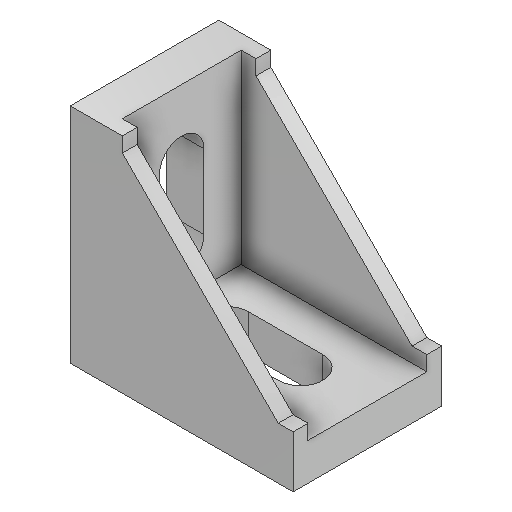
# Autodesk Inventor part: Esquinero
Saved by Autodesk Inventor 2026.1 (Build 301233000, 233)
## iProperties
Created: 2025-06-30
Part Number: Esquinero
Material: Aluminio 6061
Document SubType Name: Modeling
Designer: piero
Density: 2.7 g/cm^3
Appearance: Satinado - Plateado
Author: piero
Autodesk Inventor part; units mm, degrees
ref_plane "YZ Plane" through (0, 0, 0) normal (1, 0, 0) x (0, 1, 0)
ref_plane "XZ Plane" through (0, 0, 0) normal (0, 1, 0) x (-1, 0, 0)
ref_plane "XY Plane" through (0, 0, 0) normal (0, 0, 1) x (1, 0, 0)
sketch "Boceto1" plane through (0, 0, 0) normal (1, 0, 0) x (0, 1, 0)
  line L0 (0, 0) -> (30, 0)
  line L1 (30, 0) -> (30, -20)
  line L2 (30, -20) -> (0, -20)
  line L3 (0, -20) -> (0, 0)
  line L4 (21, -10) -> (11, -10) construction
  line L5 (21, -7) -> (11, -7)
  line L6 (11, -13) -> (21, -13)
  arc A0 (21, -13) -> (21, -7) centre (21, -10) ccw
  arc A1 (11, -7) -> (11, -13) centre (11, -10) ccw
  point P0 (16, -10)
  point P1 (24, -10)
  point P2 (30, -10)
  point P3 (0, -10)
  point P4 (8, -10)
  dimension "d0" = 30
  dimension "d1" = 20
  dimension "d2" = 10
  dimension "d3" = 6
  dimension "d4" = 6
  constraints: 16 end point, 6 point on circle, 4 tangent, 3 midpoint, 3 parallel, 2 centre point, 2 horizontal, 1 perpendicular
  measures "d0" distance of L1.end L2.end
  measures "d1" distance of L0.end L1.end
  measures "d2" distance of L4.start L4.end
  measures "d3" diameter of A1
  measures "d4" distance of point (24, -10) point (30, -10)
extrude "Extrusión1" add sketch "Boceto1" along normal blind 5
sketch "Boceto2" plane through (5, 0, 0) normal (1, 0, 0) x (0, 0, -1)
  line L0 (0, 0) -> (20, 0) projected
  line L1 (0, 0) -> (20, 0)
  line L2 (20, 0) -> (20, 5)
  line L3 (20, 5) -> (0, 5)
  line L4 (0, 5) -> (0, 0)
  dimension "d8" = 20
  dimension "d9" = 5
  constraints: 8 end point, 2 parallel, 1 horizontal, 1 perpendicular
  measures "d8" distance of L3.end L2.end
  measures "d9" distance of L2.end L1.end
extrude "Extrusión2" add sketch "Boceto2" along normal blind 25
sketch "Boceto3" plane through (5, 5, 0) normal (0, 1, 0) x (1, 0, 0)
  line L0 (6, 10) -> (16, 10) construction
  line L1 (6, 7) -> (16, 7)
  line L2 (16, 13) -> (6, 13)
  arc A0 (6, 13) -> (6, 7) centre (6, 10) ccw
  arc A1 (16, 7) -> (16, 13) centre (16, 10) ccw
  line L3 (25, 20) -> (25, 0) projected
  line L4 (0, 0) -> (25, 0) projected
  point P0 (-5, 0)
  point P1 (11, 10)
  point P2 (25, 10)
  point P3 (19, 10)
  dimension "d12" = 10
  dimension "d13" = 6
  dimension "d14" = 6
  dimension "d15" = 10
  constraints: 8 end point, 5 point on circle, 4 tangent, 2 centre point, 2 midpoint, 1 horizontal, 1 parallel
  measures "d12" distance of L0.start L0.end
  measures "d13" diameter of A1
  measures "d14" distance of point (25, 10) point (19, 10)
  measures "d15" distance from line of L4 point (11, 10)
extrude "Extrusión3" cut sketch "Boceto3" against normal blind 5
sketch "Boceto4" plane through (0, 0, 0) normal (0, 0, 1) x (1, 0, 0)
  line L0 (5, 30) -> (5, 5) projected
  line L1 (5, 5) -> (30, 5) projected
  line L2 (5, 5) -> (5, 28)
  line L3 (5, 30) -> (7, 30)
  line L4 (7, 30) -> (7, 28)
  line L5 (30, 5) -> (30, 7)
  line L6 (30, 7) -> (28, 7)
  line L7 (28, 7) -> (7, 28)
  point P0 (0, 0)
  point P1 (28, 5)
  dimension "d18" = 2
  dimension "d19" = 2
  dimension "d22" = 2
  constraints: 12 end point, 3 perpendicular, 2 point on line, 1 horizontal, 1 vertical
  measures "d18" distance of L2.end L0.start
  measures "d19" distance of point (28, 5) L1.end
  measures "d22" distance of L1.end L5.end
extrude "Extrusión4" add sketch "Boceto4" against normal blind 2
sketch "Boceto5" plane through (0, 0, -20) normal (0, 0, -1) x (-1, 0, 0)
  line L0 (-30, 0) -> (-30, 5) projected
  line L1 (-30, 0) -> (-30, 7) projected
  line L2 (-30, 5) -> (-30, 7)
  line L3 (-30, 7) -> (-28, 7)
  line L4 (-7, 30) -> (-7, 28) projected
  line L5 (-28, 7) -> (-7, 28)
  line L6 (-7, 28) -> (-7, 30)
  line L7 (-7, 30) -> (-5, 30)
  line L8 (-5, 30) -> (-5, 5)
  line L9 (-5, 5) -> (-30, 5)
  point P0 (0, 0)
  dimension "d23" = 2
  constraints: 14 end point, 4 perpendicular, 1 collinear, 1 point on line, 1 vertical
  measures "d23" distance of L1.end L3.end
extrude "Extrusión5" add sketch "Boceto5" against normal blind 2
